6f66c0c9-0f35-4514-8d5a-5b800bdad21f (Autodesk Fusion 360 design; units mm, degrees)
Autodesk Fusion 360 part; units mm, degrees
note: some values were not read from the file. Set by a fixed rule: which sketch regions a step uses.
sketch "Sketch1" plane through (0, 0, 0) normal (0, 1, 0) x (1, 0, 0)
  circle A0 centre (0, 0) radius 4.7625
  circle A1 centre (0, 0) radius 5.588
  circle A2 centre (0, 0) radius 3.9688
  circle A3 centre (0, 0) radius 4.4753
  arc A4 (5.5737, -0.3998) -> (-5.1218, -2.2344) centre (0, 0) ccw
  circle A5 centre (0, 0) radius 0.3969
  line L0 (0, 0) -> (5.588, 0) construction
  line L1 (0, 0) -> (-0.39, -4.4583)
  line L2 (0, 0) -> (-0.7771, -4.4073)
  line L3 (0, 0) -> (-1.1583, -4.3228)
  line L4 (0, 0) -> (-1.5306, -4.2054)
  line L5 (0, 0) -> (-1.8913, -4.056)
  line L6 (0, 0) -> (-2.2376, -3.8757)
  line L7 (0, 0) -> (-2.5669, -3.6659)
  line L8 (-0.39, -4.4583) -> (-0.001, -4.4923) construction
  line L9 (-0.7771, -4.4073) -> (-0.0079, -4.5429) construction
  line L10 (-1.1583, -4.3228) -> (-0.0266, -4.626) construction
  line L11 (-1.5306, -4.2054) -> (-0.0627, -4.7397) construction
  line L12 (-1.8913, -4.056) -> (-0.1216, -4.8812) construction
  line L13 (-2.2376, -3.8757) -> (-0.2083, -5.0473) construction
  line L14 (-2.5669, -3.6659) -> (-0.3275, -5.234) construction
  line L15 (0, 0) -> (-2.8767, -3.4283)
  line L16 (-2.8767, -3.4283) -> (-0.4833, -5.4366) construction
  line L17 (0, 0) -> (-3.1645, -3.1645)
  line L18 (-3.1645, -3.1645) -> (-0.6791, -5.6499) construction
  spline S0 degree 5 poles (-0.6791, -5.6499) (-0.6718, -5.6425) (-0.6572, -5.6278) (-0.6358, -5.6058) (-0.6077, -5.5764) (-0.5737, -5.5398) (-0.5407, -5.5033) (-0.5087, -5.4668) (-0.4778, -5.4304) (-0.448, -5.3941) (-0.4192, -5.3579) (-0.3914, -5.3219) (-0.3647, -5.2861) (-0.339, -5.2506) (-0.3144, -5.2153) (-0.2907, -5.1804) (-0.2682, -5.1458) (-0.2466, -5.1116) (-0.226, -5.0778) (-0.2065, -5.0445) (-0.1879, -5.0116) (-0.1704, -4.9793) (-0.1538, -4.9475) (-0.1382, -4.9164) (-0.1236, -4.8859) (-0.1099, -4.8561) (-0.0971, -4.827) (-0.0853, -4.7986) (-0.0743, -4.7711) (-0.0643, -4.7445) (-0.0551, -4.7187) (-0.0467, -4.6939) (-0.0392, -4.6701) (-0.0324, -4.6474) (-0.0264, -4.6258) (-0.0211, -4.6054) (-0.0165, -4.5862) (-0.0126, -4.5682) (-0.0094, -4.5516) (-0.0067, -4.5364) (-0.0046, -4.5227) (-0.003, -4.5105) (-0.0018, -4.5) (-0.0009, -4.4912) (-0.0002, -4.4843) (0.0001, -4.4792) (0.0002, -4.4767) (0.0002, -4.4757) (0.0001, -4.4753) (0, -4.4753) knots 0 0 0 0 0 0 0.022222 0.044444 0.066667 0.088889 0.111111 0.133333 0.155556 0.177778 0.2 0.222222 0.244444 0.266667 0.288889 0.311111 0.333333 0.355556 0.377778 0.4 0.422222 0.444444 0.466667 0.488889 0.511111 0.533333 0.555556 0.577778 0.6 0.622222 0.644444 0.666667 0.688889 0.711111 0.733333 0.755556 0.777778 0.8 0.822222 0.844444 0.866667 0.888889 0.911111 0.933333 0.955556 0.977778 1 1 1 1 1 1
  line L19 (-0.7887, -5.76) -> (-0.5695, -5.5398)
  line L20 (0.0093, -4.4845) -> (-0.0093, -4.466)
  line L21 (-0.071, -4.762) -> (0, 0)
  line L22 (0, 0) -> (-0.8866, -6.0377) construction
  line L23 (0, -4.4753) -> (0, 0) construction
  spline S1 degree 5 poles (0, -4.4753) (0, -4.4464) (0, -4.3917) (0, -4.3194) (0, -4.2389) (0, -4.1521) (0, -4.0836) (0, -4.0283) (0, -3.989) (0, -3.9688) knots 0 0 0 0 0 0 0.2 0.4 0.6 0.8 1 1 1 1 1 1
  spline S2 degree 5 poles (-1.2866, -4.2864) (-1.2783, -4.2587) (-1.2626, -4.2063) (-1.2418, -4.137) (-1.2186, -4.0599) (-1.1937, -3.9768) (-1.174, -3.9112) (-1.1581, -3.8583) (-1.1468, -3.8206) (-1.141, -3.8012) knots 0 0 0 0 0 0 0.2 0.4 0.6 0.8 1 1 1 1 1 1
  line L24 (0, -4.549) -> (0, -4.4015)
  line L25 (0, -4.0204) -> (0, -3.9171)
  line L26 (-1.3078, -4.357) -> (-1.2654, -4.2157)
  line L27 (-1.1558, -3.8507) -> (-1.1261, -3.7517)
  spline S3 degree 5 poles (-0.9739, -5.6066) (-0.9788, -5.5975) (-0.9884, -5.5792) (-1.0027, -5.5519) (-1.0211, -5.5157) (-1.0432, -5.4709) (-1.0643, -5.4264) (-1.0844, -5.3822) (-1.1035, -5.3385) (-1.1217, -5.2951) (-1.1389, -5.2522) (-1.1551, -5.2098) (-1.1704, -5.1678) (-1.1848, -5.1264) (-1.1983, -5.0855) (-1.2108, -5.0453) (-1.2225, -5.0056) (-1.2334, -4.9667) (-1.2433, -4.9284) (-1.2525, -4.8909) (-1.2608, -4.8541) (-1.2683, -4.8181) (-1.275, -4.7829) (-1.281, -4.7486) (-1.2863, -4.7151) (-1.2908, -4.6826) (-1.2947, -4.6511) (-1.2979, -4.6206) (-1.3004, -4.5911) (-1.3024, -4.5626) (-1.3038, -4.5353) (-1.3047, -4.5092) (-1.3051, -4.4842) (-1.305, -4.4605) (-1.3046, -4.4381) (-1.3038, -4.417) (-1.3026, -4.3973) (-1.3012, -4.379) (-1.2996, -4.3622) (-1.2977, -4.3468) (-1.2958, -4.3331) (-1.2938, -4.3209) (-1.292, -4.3105) (-1.2904, -4.3019) (-1.289, -4.295) (-1.2879, -4.2901) (-1.2872, -4.2876) (-1.2869, -4.2867) (-1.2867, -4.2864) (-1.2866, -4.2864) knots 0 0 0 0 0 0 0.022222 0.044444 0.066667 0.088889 0.111111 0.133333 0.155556 0.177778 0.2 0.222222 0.244444 0.266667 0.288889 0.311111 0.333333 0.355556 0.377778 0.4 0.422222 0.444444 0.466667 0.488889 0.511111 0.533333 0.555556 0.577778 0.6 0.622222 0.644444 0.666667 0.688889 0.711111 0.733333 0.755556 0.777778 0.8 0.822222 0.844444 0.866667 0.888889 0.911111 0.933333 0.955556 0.977778 1 1 1 1 1 1
  line L28 (-0.9006, -5.7436) -> (-1.0472, -5.4697)
  line L29 (-1.2982, -4.2925) -> (-1.2751, -4.2802)
  point P0 (-0.071, -4.762)
  point P1 (0, -3.9688)
  point P2 (-1.1001, -5.346)
  point P3 (-1.191, -5.1072)
  point P4 (-1.2515, -4.8941)
  point P5 (-1.2869, -4.7101)
  point P6 (-1.3026, -4.5576)
  point P7 (-1.3045, -4.4384)
  point P8 (-1.2985, -4.3534)
  point P9 (-1.2905, -4.3029)
  point P10 (-1.141, -3.8012)
  dimension "d2" = 11.176
  dimension "id" = 7.9375
  dimension "BaseDiameter" = 8.9506
  dimension "d1" = 0.7937
  dimension "d34" = 5
  dimension "d35" = 5
  dimension "d36" = 5
  dimension "d37" = 5
  dimension "d38" = 5
  dimension "d39" = 5
  dimension "d41" = 0.3905
  dimension "d42" = 0.7811
  dimension "d43" = 1.1716
  dimension "d44" = 1.5622
  dimension "d45" = 1.9527
  dimension "d46" = 2.3433
  dimension "d47" = 2.7338
  dimension "d48" = 5
  dimension "d49" = 3.1243
  dimension "d50" = 5
  dimension "d51" = 3.5149
  dimension "d55" = 7.5
  dimension "d60" = 5
  constraint coincident A0.centre A1.centre
  constraint concentric A0 A2
  constraint coincident A1 A4.end
  constraint horizontal L0
  constraint coincident A4 L0.end
  constraint coincident A3 S0.end
  constraint coincident A3 L1.end
  constraint coincident A3 L2.end
  constraint coincident A3 L3.end
  constraint coincident A3 L4.end
  constraint coincident A3 L5.end
  constraint coincident A3 L6.end
  constraint coincident A3 L7.end
  constraint vertical A0.centre S0.end
  constraint tangent A3 L8
  constraint tangent A3 L9
  constraint tangent A3 L10
  constraint tangent A3 L11
  constraint tangent A3 L12
  constraint tangent A3 L13
  constraint tangent A3 L14
  constraint coincident A3 L15.end
  constraint tangent A3 L16
  constraint coincident A3 L17.end
  constraint tangent A3 L18
  constraint midpoint L18.end L19
  constraint midpoint S0.end L20
  constraint coincident A0 P0
  constraint coincident S0 P0
  constraint coincident P0 L21.start
  constraint coincident L23 P1
  constraint coincident A2 P1
  constraint coincident P1 S1.end
  constraint midpoint S0.end L24
  constraint midpoint P1 L25
  constraint symmetric S0.end L22 S2.start
  constraint symmetric L8.end L22 P9
  constraint symmetric L9.end L22 P8
  constraint symmetric L10.end L22 P7
  constraint symmetric L11.end L22 P6
  constraint symmetric L12.end L22 P5
  constraint symmetric L13.end L22 P4
  constraint symmetric L14.end L22 P3
  constraint symmetric L16.end L22 P2
  constraint symmetric L18.end L22 S3.start
  constraint symmetric L19.start L22 L28.start
  constraint symmetric L19.end L22 L28.end
  constraint symmetric L20.start L22 L29.start
  constraint symmetric L20.end L22 L29.end
  constraint symmetric L22 P1 P10
  constraint symmetric L22 L24.start L26.start
  constraint symmetric L22 L24.end L26.end
  constraint symmetric L22 L25.start L27.start
  constraint symmetric L22 L25.end L27.end
  constraint vertical L24
  constraint vertical L25
  measures "d2" diameter of A1
  measures "id" diameter of A2
  measures "BaseDiameter" diameter of A3
  measures "d1" diameter of A5
  measures "d34" angle of L1 L2
  measures "d35" angle of L2 L3
  measures "d36" angle of L3 L4
  measures "d37" angle of L4 L5
  measures "d38" angle of L5 L6
  measures "d39" angle of L6 L7
  measures "d41" distance of L1.end L8.end
  measures "d42" distance of L2.end L9.end
  measures "d43" distance of L3.end L10.end
  measures "d44" distance of L4.end L11.end
  measures "d45" distance of L5.end L12.end
  measures "d46" distance of L6.end L13.end
  measures "d47" distance of L7.end L14.end
  measures "d48" angle of L7 L15
  measures "d49" distance of L15.end L16.end
  measures "d50" angle of L15 L17
  measures "d51" distance of L17.end L18.end
  measures "d55" angle of L21 L22
  measures "d60" angle of L1 L23
extrude "Extrude1" add sketch "Sketch1" along normal blind 304.8 contours A0 A1 S0 S3 | A3 S0 L21 | A0 A3 L21 S3 | A2 A3 L21 S1 L24 L25 | A2 A3 L1 L21 | A2 A3 L3 S2 L26 L27 | A2 A3 L1 L2 | A2 A3 L2 L3 makes body 1
pattern_circular "C-Pattern2" count 12 over 360 about axis through (0, 1.75, 0) along (0, 1, 0) of bodies 1 makes body 2 at (1.7576, 203.2, 3.5583) makes body 3 at (3.3013, 203.2, 2.2028) makes body 4 at (3.9604, 203.2, 0.257) makes body 5 at (3.4995, 203.2, -1.872) makes body 6 at (2.2028, 203.2, -3.3013) makes body 7 at (0.257, 203.2, -3.9604) makes body 8 at (-1.7576, 203.2, -3.5583) makes body 9 at (-3.3013, 203.2, -2.2028) makes body 10 at (-3.9604, 203.2, -0.257) makes body 11 at (-3.5583, 203.2, 1.7576) makes body 12 at (-2.2028, 203.2, 3.3013)
extrude "Extrude2" add sketch "Sketch1" along normal blind 304.8 contours A2 A5 L17 L21 | A2 A5 L1 L21 | A2 A5 L1 L2 | A2 A5 L3 L4 | A2 A5 L4 L5 | A2 A5 L2 L3 | A2 A5 L15 L17 | A2 A5 L5 L6 | A2 A5 L7 L15 | A2 A5 L6 L7 bodies 1 2 3 4 5 6 7 8 9 10 11 12
ref_plane "WorkPlane1" through (6.2747, 152.4, -0.8261) normal (0.130526, 0, 0.991445) x (0.991445, 0, -0.130526)
fillet "Fillet1" [suppressed]
mirror "Mirror3" [suppressed]
pattern_circular "C-Pattern1" [suppressed]
equation "d = 0.375 in"
equation "OutsideDiameter = d2"
equation "PitchDiameter = d"
equation "id = PitchDiameter - 2 * ( PitchDiameter / TeethNumber )"
equation "BaseDiameter = PitchDiameter * cos(20 deg)"
equation "Length = 12 in"
equation "t = 12"
equation "ShaftDiameter = d1"
equation "TeethNumber = t"
equation "Pitch = 32"
equation "d30 = ( 1.25 * ( PitchDiameter / TeethNumber ) ) - ( PitchDiameter / TeethNumber )"
equation "Basecircum = PI * PitchDiameter * cos(20 deg)"
equation "d41 = Basecircum * 5 / 360"
equation "d42 = Basecircum * 10 / 360"
equation "d43 = Basecircum * 15 / 360"
equation "d44 = Basecircum * 20 / 360"
equation "d45 = Basecircum * 25 / 360"
equation "d46 = Basecircum * 30 / 360"
equation "d47 = Basecircum * 35 / 360"
equation "d49 = Basecircum * 40 / 360"
equation "d51 = Basecircum * 45 / 360"
equation "d55 = ( 360 / ( 4 * TeethNumber ) ) * 1 deg"
